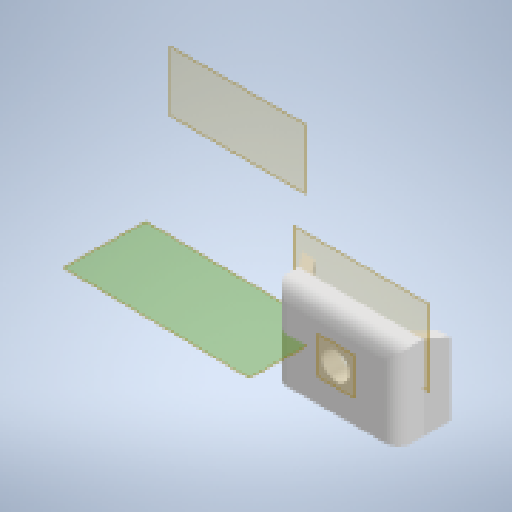
# Autodesk Inventor part: крышка камера
Saved by Autodesk Inventor 2024.2 (Build 282272000, 272)
## iProperties
Created: 2025-10-05
Part Number: крышка камера
Material: PLA
Document SubType Name: Modeling
Designer: katya_notebook
Density: 1.24 g/cm^3
Appearance: Типовые
Author: katya_notebook
Autodesk Inventor part; units mm, degrees
ref_plane "YZ Plane" through (0, 0, 0) normal (1, 0, 0) x (0, 1, 0)
ref_plane "XZ Plane" through (0, 0, 0) normal (0, 1, 0) x (-1, 0, 0)
ref_plane "XY Plane" through (0, 0, 0) normal (0, 0, 1) x (1, 0, 0)
ref_plane "РабПлоскость1" through (0, 97.1605, 0) normal (0, 0, 1) x (-1, 0, 0)
ref_plane "РабПлоскость8" through (0, 0, 0) normal (0, 0, 1) x (1, 0, 0)
sketch "Эскиз20" plane through (0, 0, 0) normal (0, 0, 1) x (1, 0, 0)
  point P0 (0, 0)
sketch "Эскиз1" plane through (0, 97.1605, 0) normal (0, 0, 1) x (-1, 0, 0)
  line L0 (53.6991, 17.5343) -> (19.6991, 17.5343) projected
  line L1 (0.5009, 79.3291) -> (0.5009, 123.8405)
  line L2 (0.5009, 123.8405) -> (-73.8991, 123.8405)
  line L3 (-73.8991, 79.3291) -> (-73.8991, 123.8405)
  line L4 (0.5009, 79.3291) -> (0.5009, 73.8405)
  line L5 (-73.8991, 79.3291) -> (-73.8991, 73.8405)
  line L6 (-73.8991, 73.8405) -> (0.5009, 73.8405)
  line L7 (-73.3991, 110.6606) -> (-73.3991, 83.6606) projected
  line L8 (-73.8991, 123.8405) -> (0.5009, 123.8405) projected
  dimension "d55" = 0
  dimension "d56" = 50
  dimension "d57" = 0
  dimension "d58" = 0
  constraints: 12 end point, 2 perpendicular, 1 horizontal, 1 vertical
  measures "d55" distance between parallel lines of L8 L2
  measures "d56" distance between parallel lines of L6 L2
  measures "d57" distance from line of L3 L8.start
  measures "d58" distance of L1.end L8.end
extrude "Выдавливание1" add sketch "Эскиз1" along normal blind 15
ref_plane "РабПлоскость9" through (36.6991, -1.4657, 15) normal (0, 0, 1) x (1, 0, 0)
sketch "Эскиз4" plane through (36.6991, -1.4657, 15) normal (0, 0, 1) x (1, 0, 0)
  circle A0 centre (0, 0) radius 8
  point P0 (-36.6991, 1.4657)
  dimension "d8" = 16
  constraints: 1 centre point
  measures "d8" diameter of A0
extrude "Выдавливание3" cut sketch "Эскиз4" against normal blind 15
sketch "Эскиз5" plane through (0, 97.1605, 0) normal (0, 0, 1) x (-1, 0, 0)
  circle A0 centre (36.6991, -1.4657) radius 8 projected
  line L0 (-57.6991, 119.6262) -> (-15.6991, 119.6262)
  line L1 (-15.6991, 119.6262) -> (-15.6991, 77.6262)
  line L2 (-15.6991, 77.6262) -> (-57.6991, 77.6262)
  line L3 (-57.6991, 77.6262) -> (-57.6991, 119.6262)
  line L4 (-57.6991, 119.6262) -> (-15.6991, 77.6262) construction
  line L5 (-15.6991, 119.6262) -> (-57.6991, 77.6262) construction
  point P0 (-36.6991, 98.6262)
  dimension "d65" = 42
  dimension "d66" = 42
  constraints: 12 end point, 2 midpoint, 2 parallel, 1 horizontal, 1 perpendicular
  measures "d65" distance of L1.end L2.end
  measures "d66" distance of L0.end L1.end
extrude "Выдавливание4" cut sketch "Эскиз5" along normal blind 5 contours L0 L1 L2 L3
ref_plane "РабПлоскость2" through (-83.6534, 0, 27.511) normal (0, -1, 0) x (0.9999139, 0, 0.0131203)
sketch "Эскиз7" plane through (-83.6534, 23.32, 27.511) normal (0, -1, 0) x (0.9999139, 0, 0.0131203)
  line L0 (79.6013, -33.3861) -> (83.2852, -28.6062) projected
  line L1 (79.5461, -37.5999) -> (79.6013, -33.3861) projected
  line L2 (75.3464, -37.5448) -> (79.5461, -37.5999) projected
  line L3 (75.3464, -37.5448) -> (83.3464, -37.5448)
  line L4 (83.3464, -37.5448) -> (90.6981, -28.7034)
  line L5 (157.178, -29.5757) -> (82.7844, -28.5996) projected
  line L6 (83.2852, -28.6062) -> (90.6981, -28.7034)
  line L7 (82.7844, -28.5996) -> (75.3464, -37.5448)
  line L8 (157.3748, -14.577) -> (82.9812, -13.6009) projected
  line L9 (120.178, -14.089) -> (119.9812, -29.0877)
  line L10 (160.2344, -34.4441) -> (156.6772, -29.5692)
  line L11 (160.1791, -38.6579) -> (160.2344, -34.4441)
  line L12 (164.3787, -38.713) -> (160.1791, -38.6579)
  line L13 (164.3787, -38.713) -> (156.3815, -38.5031)
  line L14 (156.3815, -38.5031) -> (149.2644, -29.4719)
  line L15 (156.6772, -29.5692) -> (149.2644, -29.4719)
  line L16 (157.178, -29.5757) -> (164.3787, -38.713)
  dimension "d67" = 8
  constraints: 24 end point, 6 symmetric about line, 2 midpoint, 1 collinear, 1 horizontal, 1 parallel, 1 point on line
  measures "d67" distance of L2.start L3.end
ref_plane "РабПлоскость3" through (-3.0009, -24.18, -16.4278) normal (0.7071068, 0.7071068, 0) x (-0.7071068, 0.7071068, 0)
ref_plane "РабПлоскость10" through (-2.8403, -24.3405, -16.5539) normal (0.7071068, 0.7071068, 0) x (-0.7071068, 0.7071068, 0)
extrude "Выдавливание6" add sketch "Эскиз7" against normal up to surface contours L1 L3 L7 L5 L0 | L0 L5 L4 L3 L1 surface through (-2.8403, -24.3405, -16.5539) normal (0.7071068, 0.7071068, 0)
sketch "Эскиз21" plane through (-0.5009, 23.32, 15) normal (0, 1, 0) x (1, 0, 0)
  line L0 (73.7207, 23.9371) -> (66.4857, 15) projected
  line L1 (81.72, 24.042) -> (73.7207, 23.9371) projected
  line L2 (74.4, 15) -> (81.72, 24.042) projected
  line L3 (74.4, 15) -> (7.9143, 15) projected
  point P0 (0.5009, 15)
ref_plane "РабПлоскость11" through (73.6907, -26.8885, -16.5539) normal (-0.7071068, 0.7071068, 0) x (0, 0, 1)
extrude "Выдавливание18" add sketch "Эскиз21" against normal up to surface surface through (73.6907, -26.8885, -16.5539) normal (-0.7071068, 0.7071068, 0)
sketch "Эскиз22" plane through (0, 97.1605, 15) normal (0, 0, 1) x (1, 0, 0)
  line L0 (-5.7, -123.8405) -> (75.0013, -123.8405)
  line L1 (75.0013, -123.8405) -> (75.0013, -145.8361)
  line L2 (75.0013, -145.8361) -> (-5.7, -145.8361)
  line L3 (-5.7, -145.8361) -> (-5.7, -123.8405)
  point P0 (0, -97.1605)
  constraints: 8 end point, 2 parallel, 1 horizontal, 1 perpendicular
extrude "Выдавливание19" cut sketch "Эскиз22" against normal blind 107.5
ref_plane "РабПлоскость4" through (-83.6534, 0, 27.511) normal (0, -1, 0) x (0.9999139, 0, 0.0131203)
ref_plane "РабПлоскость5" through (73.8991, -26.68, -16.4278) normal (-0.7071068, 0.7071068, 0) x (0, 0, 1)
fillet "Сопряжение2" radius 8 3 edges at (-0.5009, -1.68, 15) (36.6991, 23.32, 15) (73.8991, -1.68, 15)
sketch "Эскиз9" plane through (0, 97.1605, 5) normal (0, 0, -1) x (1, 0, 0)
  circle A0 centre (36.6991, 98.6262) radius 8 projected
  circle A1 centre (36.6991, 98.6262) radius 8
  line L0 (51.1991, 84.1262) -> (22.1991, 84.1262)
  line L1 (22.1991, 84.1262) -> (22.1991, 113.1262)
  line L2 (22.1991, 113.1262) -> (51.1991, 113.1262)
  line L3 (51.1991, 113.1262) -> (51.1991, 84.1262)
  line L4 (51.1991, 84.1262) -> (22.1991, 113.1262) construction
  line L5 (22.1991, 84.1262) -> (51.1991, 113.1262) construction
  circle A2 centre (22.1991, 113.1262) radius 2.1
  circle A3 centre (22.1991, 84.1262) radius 2.1
  circle A4 centre (51.1991, 113.1262) radius 2.1
  circle A5 centre (51.1991, 84.1262) radius 2.1
  point P0 (0, 97.1605)
  point P1 (-36.6991, -1.4657)
  dimension "d72" = 29
  dimension "d73" = 4.2
  dimension "d74" = 0
  dimension "d75" = 0
  constraints: 12 end point, 5 centre point, 4 coincident, 3 equal radius, 2 midpoint, 2 parallel, 2 perpendicular, 1 horizontal
  measures "d72" distance of L1.end L2.end
  measures "d73" diameter of A5
  measures "d74" distance of A0.centre A1.centre
  measures "d75" distance of A0.centre A1.centre
extrude "Выдавливание8" cut sketch "Эскиз9" against normal blind 5 contours A3 L1 L0 | L0 L1 A3 | A5 L3 L0 | L0 L3 A5 | A2 L2 L1 | L1 L2 A2 | A4 L2 L3 | L3 L2 A4
chamfer "Фаска1" distance 2 angle 45 2 edges at (7.4135, -1.68, 0) (65.9848, -1.68, 0)
sketch "Эскиз11" plane through (0, 97.1605, 0) normal (0, 0, -1) x (1, 0, 0)
  spline S0 degree 3 poles (67.1991, 94.4586) (67.2707, 94.5756) (67.3559, 94.6822) (67.6001, 94.9261) (67.7927, 95.0571) (68.2121, 95.2296) (68.4388, 95.2712) (68.8685, 95.2712) (69.0994, 95.2264) (69.5211, 95.0484) (69.712, 94.9154) (70.0075, 94.6141) (70.135, 94.427) (70.3059, 94.0132) (70.3491, 93.7862) (70.3491, 93.3563) (70.3059, 93.1293) (70.135, 92.7154) (70.0075, 92.5284) (69.712, 92.227) (69.5211, 92.094) (69.0994, 91.916) (68.8685, 91.8712) (68.4388, 91.8712) (68.2121, 91.9128) (67.7927, 92.0853) (67.6001, 92.2164) (67.3559, 92.4602) (67.2707, 92.5668) (67.1991, 92.6838) knots 0.089167 0.089167 0.089167 0.089167 0.128222 0.128222 0.192735 0.192735 0.257248 0.257248 0.324519 0.324519 0.391791 0.391791 0.456277 0.456277 0.520762 0.520762 0.585248 0.585248 0.649734 0.649734 0.717005 0.717005 0.784277 0.784277 0.84879 0.84879 0.913303 0.913303 0.952358 0.952358 0.952358 0.952358 projected
  arc A0 (67.1991, 94.4586) -> (67.1991, 92.6838) centre (68.6491, 93.5712) ccw projected
  spline S1 degree 3 poles (6.1991, 92.5251) (6.1554, 92.469) (6.1087, 92.4165) (5.9081, 92.2163) (5.7158, 92.0854) (5.2966, 91.9129) (5.0698, 91.8712) (4.6402, 91.8712) (4.4096, 91.9159) (3.9883, 92.0934) (3.7975, 92.2261) (3.5015, 92.5273) (3.3736, 92.7148) (3.2024, 93.1292) (3.1591, 93.3563) (3.1591, 93.5712) (3.1591, 93.7861) (3.2024, 94.0132) (3.3736, 94.4276) (3.5015, 94.6151) (3.7975, 94.9163) (3.9883, 95.049) (4.4096, 95.2266) (4.6402, 95.2712) (5.0698, 95.2712) (5.2966, 95.2295) (5.7158, 95.057) (5.9081, 94.9261) (6.1087, 94.7259) (6.1554, 94.6734) (6.1991, 94.6173) knots -0.412165 -0.412165 -0.412165 -0.412165 -0.391556 -0.391556 -0.327162 -0.327162 -0.262769 -0.262769 -0.195855 -0.195855 -0.128941 -0.128941 -0.06447 -0.06447 0 0 0 0.06447 0.06447 0.128941 0.128941 0.195855 0.195855 0.262769 0.262769 0.327162 0.327162 0.391556 0.391556 0.412165 0.412165 0.412165 0.412165 projected
  arc A1 (6.1991, 92.5251) -> (6.1991, 94.6173) centre (4.8591, 93.5712) ccw projected
  circle A2 centre (68.6491, 93.5712) radius 2.1
  circle A3 centre (4.8591, 93.5712) radius 2.1
  point P0 (0, 97.1605)
  dimension "d81" = 4.2
  dimension "d82" = 4.2
  constraints: 2 centre point, 2 coincident
  measures "d81" diameter of A2
  measures "d82" diameter of A3
extrude "Выдавливание10" cut sketch "Эскиз11" along normal blind 20 and the other way blind 20 contours S0 A0 | S1 A1
ref_plane "РабПлоскость6" through (-16.7083, 0, -45.6496) normal (0, -1, 0) x (1, 0, 0)
ref_plane "РабПлоскость7" through (-14.5982, 0, -45.6496) normal (0, -1, 0) x (1, 0, 0)
